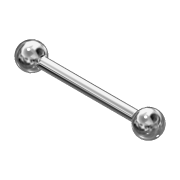
# Autodesk Inventor part: Prop_Conrod
Saved by Autodesk Inventor 2022 Beta2 (Build 260130000, 130) ContinuousBuild 0
## iProperties
Created: 2013-03-11
Part Number: Prop_Conrod
Material: Nickel-Copper Alloy 400
Document SubType Name: Modeling
Designer: user
Density: 8.83 g/cm^3
Mass: 426.06 g
Surface Area: 108.721 cm^2
Volume: 48.2514 cm^3
Appearance: Chrome - Polished
Author: user
Autodesk Inventor part; units mm, degrees
ref_plane "YZ Plane" through (0, 0, 0) normal (1, 0, 0) x (0, 1, 0)
ref_plane "XZ Plane" through (0, 0, 0) normal (0, 1, 0) x (-1, 0, 0)
ref_plane "XY Plane" through (0, 0, 0) normal (0, 0, 1) x (1, 0, 0)
sketch "Sketch1" plane through (0, 0, 0) normal (0, 0, 1) x (1, 0, 0)
  circle A0 centre (0, 0) radius 15.748
  circle A1 centre (152.4, 0) radius 15.748
  line L0 (0, 0) -> (152.4, 0)
  line L1 (0, 15.748) -> (0, -15.748)
  line L2 (152.4, 15.748) -> (152.4, -15.748)
  dimension "d2" = 15.748
  dimension "d4" = 152.4
  constraints: 6 end point, 4 point on circle, 2 centre point, 1 coincident, 1 equal radius, 1 horizontal, 1 parallel, 1 perpendicular
  measures "d2" radius of A0
  measures "d4" distance of L0.end L0.start
revolve "Revolution1" add sketch "Sketch1" angle 360 about axis through (0, 15.748, 0) along (0, -1, 0) contours L1 A0
revolve "Revolution2" add sketch "Sketch1" angle 360 about axis through (152.4, 15.748, 0) along (0, -1, 0) contours A1 L2 L0 | L0 L2 A1
sketch "Sketch2" plane through (0, 0, 0) normal (1, 0, 0) x (0, 1, 0)
  circle A0 centre (0, 0) radius 6.35
  dimension "d7" = 12.7
  constraints: 1 centre point, 1 coincident
  measures "d7" diameter of A0
sweep "Sweep1" add profiles "Sketch2" path "Sketch1" path curves L0
fillet "Fillet1" radius 3.175 3 edges at (14.411, -6.35, 0) (137.989, 0, 6.35) (137.989, 0, -6.35)
body "Solid1"
